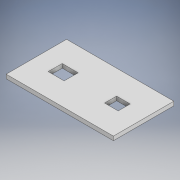
# Autodesk Inventor part: chair power plate
Saved by Autodesk Inventor 2021 (Build 250183000, 183)
## iProperties
Created: 2023-01-23
Part Number: chair power plate
Material: Generic
Document SubType Name: Modeling
Designer: boyle
Density: 1 g/cm^3
Appearance: Default
Author: boyle
Autodesk Inventor part; units mm, degrees
ref_plane "YZ Plane" through (0, 0, 0) normal (1, 0, 0) x (0, 1, 0)
ref_plane "XZ Plane" through (0, 0, 0) normal (0, 1, 0) x (-1, 0, 0)
ref_plane "XY Plane" through (0, 0, 0) normal (0, 0, 1) x (1, 0, 0)
sketch "Sketch1" plane through (0, 0, 0) normal (0, 1, 0) x (-1, 0, 0)
  line L0 (0, 0) -> (-136.144, 0)
  line L1 (-136.144, 0) -> (-136.144, -76.708)
  line L2 (-136.144, -76.708) -> (0, -76.708)
  line L3 (0, -76.708) -> (0, 0)
  line L4 (-23.9341, -47.3101) -> (-44.2537, -47.1769)
  line L5 (-44.2537, -47.1769) -> (-44.1372, -29.3973)
  line L6 (-44.1372, -29.3973) -> (-23.8176, -29.5304)
  line L7 (-23.8176, -29.5304) -> (-23.9341, -47.3101)
  line L8 (-94.2086, -30.7353) -> (-94.2453, -45.9753)
  line L9 (-94.2453, -45.9753) -> (-111.5172, -45.9338)
  line L10 (-111.5172, -45.9338) -> (-111.4806, -30.6938)
  line L11 (-111.4806, -30.6938) -> (-94.2086, -30.7353)
  line L12 (-68.072, -76.708) -> (-68.072, 0)
  line L13 (-136.144, -76.708) -> (-68.072, -76.708)
  line L14 (-102.108, -76.708) -> (-103.5543, 0)
  line L15 (-111.4806, -30.6938) -> (-94.2453, -45.9753)
  line L16 (-94.2086, -30.7353) -> (-111.5172, -45.9338)
  line L17 (-44.1372, -29.3973) -> (-23.9341, -47.3101)
  line L18 (-44.2537, -47.1769) -> (-23.8176, -29.5304)
  line L19 (-68.072, -76.708) -> (0, -76.708)
  line L20 (-34.036, -76.708) -> (-34.036, 0)
  line L21 (-68.072, -38.354) -> (0, -38.354)
  line L22 (-68.072, -38.354) -> (-136.144, -38.354)
  dimension "d0" = 136.144
  dimension "d1" = 76.708
  dimension "d2" = 20.32
  dimension "d3" = 17.78
  dimension "d4" = 15.24
  dimension "d6" = 17.272
  constraints: 46 end point, 7 midpoint, 7 parallel, 5 perpendicular, 2 point on line, 1 collinear, 1 horizontal
  measures "d0" distance of L1.end L2.end
  measures "d1" distance of L0.end L1.end
  measures "d2" distance of L4.start L4.end
  measures "d3" distance of L4.end L5.end
  measures "d4" distance of L8.start L8.end
  measures "d6" distance of L8.end L9.end
extrude "Extrusion1" add sketch "Sketch1" along normal blind 5.08 contours L3 L21 L7 L6 L20 L0 | L20 L6 L5 L21 L12 L0 | L3 L2 L20 L4 L7 L21 | L12 L22 L8 L11 L14 L0 | L14 L11 L10 L22 L1 L0 | L21 L5 L4 L20 L2 L12 | L12 L2 L14 L9 L8 L22 | L22 L10 L9 L14 L2 L1
body "Solid1"
